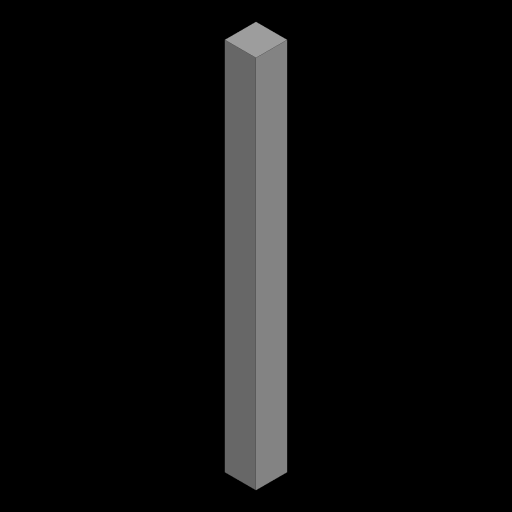
# Autodesk Inventor part: valve_mount_pin
Saved by Autodesk Inventor 2023 (Build 270158000, 158)
## iProperties
Created: 2024-07-04
Part Number: valve_mount_pin
Material: 일반
Document SubType Name: Modeling
Designer: OMS55
Density: 1 g/cm^3
Appearance: 기본값
Author: OMS55
Autodesk Inventor part; units mm, degrees
ref_plane "YZ Plane" through (0, 0, 0) normal (1, 0, 0) x (0, 1, 0)
ref_plane "XZ Plane" through (0, 0, 0) normal (0, 1, 0) x (-1, 0, 0)
ref_plane "XY Plane" through (0, 0, 0) normal (0, 0, 1) x (1, 0, 0)
sketch "스케치1" plane through (0, 0, 0) normal (0, 1, 0) x (-1, 0, 0)
  line L0 (0, 0) -> (-2.5, 0)
  line L1 (-2.5, 0) -> (-2.5, -2.5)
  line L2 (-2.5, -2.5) -> (0, -2.5)
  line L3 (0, -2.5) -> (0, 0)
  dimension "d0" = 2.5
  dimension "d1" = 2.5
  constraints: 8 end point, 2 parallel, 1 coincident, 1 horizontal, 1 perpendicular
  measures "d0" distance of L2.end L0.start
  measures "d1" distance of L1.end L2.end
extrude "돌출1" add sketch "스케치1" along normal blind 30
